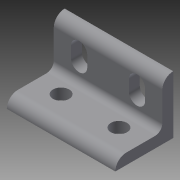
# Autodesk Inventor part: 4260
Saved by Autodesk Inventor 2014 SP2 (Build 180246200, 246)
## iProperties
Created: 2019-11-07
Part Number: 4260
Material: Generic
Catalog Web Link: www.cadenas.de
Description: 4260, 4290, 4260-Black, 4290-Black-Joining Plates - 4 Hole Slotted Inside Corner Bracket
Vendor: 8020
Document SubType Name: Modeling
Designer: psadmin
Manufacturer: 8020
Mass: 9.01421 g
Surface Area: 50.6591 cm^2
Volume: 9.01421 cm^3
Density: 1 g/cm^3
Appearance: PSOLRGB-191-191-191
Category: PARTsolutions
Company: 8020
Title: 4260
Author: Cadenas PARTsolutions
Comments: Joining Plates - 4 Hole Slotted Inside Corner Bracket
PSOL_IDENT_0: {$CADENAS_DATA\23d-libs\8020\inch\joining_plates\4260.prj},176 {VTYP=3D},{NB=4260},{LINA=4260},{NN=4
PSOL_IDENT_1: 260, 4290, 4260-Black, 4290-Black},{DATE=01.10.2019 06:04:23},{GEOMDATE=28.06.2017 15:53:00},{VERSIO
PSOL_IDENT_2: N=},{LINEID=10},{WBVAR=},{WBNUMERIC=}  {NB=4260},{LINA=4260},{KT=DUMMY},{PN=4260},{A=1.875},{B=1.000
PSOL_IDENT_3: },{C=1.000},{D=0.312},{E=0.188},{F=0.281},{W=.055},{A1=0.4375},{A2=1.437},{D1=0.188},{R=0.125},{COLO
PSOL_IDENT_4: R=.75,.75,.75}
NN: 4260, 4290, 4260-Black, 4290-Black
NT: Joining Plates - 4 Hole Slotted Inside Corner Bracket
NB: 4260
NBSYN: $PN.
LINA: 4260
PN: 4260
A: 1.875
B: 1
C: 1
D: 0.312
E: 0.188
F: 0.281
W: .055
SUPPLIER: 8020
ARTICLENO: 4260
BOMINFO: 4260
CREATOR: CADENAS GmbH
Autodesk Inventor part; units mm, degrees
ref_plane "YZ Plane" through (0, 0, 0) normal (1, 0, 0) x (0, 1, 0)
ref_plane "XZ Plane" through (0, 0, 0) normal (0, 1, 0) x (-1, 0, 0)
ref_plane "XY Plane" through (0, 0, 0) normal (0, 0, 1) x (1, 0, 0)
sketch "Sketch_1" plane through (0, 0, 0) normal (1, 0, 0) x (0, 1, 0)
  line L0 (0, 25.4) -> (0, 0)
  line L1 (0, 0) -> (25.4, 0)
  arc A0 (25.4, 0) -> (20.6248, 4.7752) centre (20.6248, 0) ccw
  line L2 (20.6248, 4.7752) -> (7.9502, 4.7752)
  arc A1 (4.7752, 7.9502) -> (7.9502, 4.7752) centre (7.9502, 7.9502) ccw
  line L3 (4.7752, 7.9502) -> (4.7752, 20.6248)
  arc A2 (4.7752, 20.6248) -> (0, 25.4) centre (0, 20.6248) ccw
  constraints: 8 end point, 6 point on circle, 3 centre point
extrude "Extrusion1" add sketch "Sketch_1" along normal mid plane 47.625
sketch "Sketch2" plane through (-23.8125, 0, 0) normal (0, -1, 0) x (1, 0, 0)
  point P0 (36.5125, 12.7)
hole "Hole1" at (12.7, 0, 12.7) direction (0, 1, 0) diameter 7.1374 depth 10.4648
sketch "Sketch3" plane through (-23.8125, 0, 0) normal (0, -1, 0) x (1, 0, 0)
  point P0 (11.1252, 12.7)
hole "Hole2" at (-12.6873, 0, 12.7) direction (0, 1, 0) diameter 7.1374 depth 10.4648
sketch "Sketch_2" plane through (0, 0, 0) normal (0, 0, 1) x (1, 0, 0)
  arc A0 (9.1313, 12.7) -> (16.2687, 12.7) centre (12.7, 12.7) ccw
  line L0 (16.2687, 12.7) -> (16.2687, 17.4752)
  arc A1 (16.2687, 17.4752) -> (9.1313, 17.4752) centre (12.7, 17.4752) ccw
  line L1 (9.1313, 17.4752) -> (9.1313, 12.7)
  constraints: 4 end point, 4 point on circle, 2 centre point
extrude "Extrusion2" cut sketch "Sketch_2" along normal blind 7.1628
sketch "Sketch_3" plane through (0, 0, 0) normal (0, 0, 1) x (1, 0, 0)
  arc A0 (-16.2687, 12.7) -> (-9.1313, 12.7) centre (-12.7, 12.7) ccw
  line L0 (-9.1313, 12.7) -> (-9.1313, 17.4752)
  arc A1 (-9.1313, 17.4752) -> (-16.2687, 17.4752) centre (-12.7, 17.4752) ccw
  line L1 (-16.2687, 17.4752) -> (-16.2687, 12.7)
  constraints: 4 end point, 4 point on circle, 2 centre point
extrude "Extrusion3" cut sketch "Sketch_3" along normal blind 7.1628
body "Solid1"
